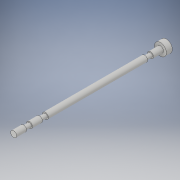
# Autodesk Inventor part: TornilloBasePixhawx
Saved by Autodesk Inventor 2019 (Build 230136000, 136)
## iProperties
Created: 2019-03-06
Part Number: TornilloBasePixhawx
Material: Generic
Document SubType Name: Modeling
Designer: Kenny
Density: 1 g/cm^3
Appearance: Default
Author: Kenny
Autodesk Inventor part; units mm, degrees
ref_plane "YZ Plane" through (0, 0, 0) normal (1, 0, 0) x (0, 1, 0)
ref_plane "XZ Plane" through (0, 0, 0) normal (0, 1, 0) x (-1, 0, 0)
ref_plane "XY Plane" through (0, 0, 0) normal (0, 0, 1) x (1, 0, 0)
sketch "Sketch1" plane through (0, 0, 0) normal (0, 0, 1) x (1, 0, 0)
  circle A0 centre (0, 0) radius 3
  dimension "d0" = 6
  constraints: 1 centre point, 1 coincident
  measures "d0" diameter of A0
extrude "Extrusion1" add sketch "Sketch1" along normal blind 3
sketch "Sketch5" plane through (0, 0, 3) normal (0, 0, 1) x (1, 0, 0)
  circle A0 centre (0, 0) radius 1.5
  dimension "d6" = 3
  constraints: 1 centre point, 1 coincident
  measures "d6" diameter of A0
extrude "Extrusion3" add sketch "Sketch5" along normal blind 5
sketch "Sketch6" plane through (0, 0, 8) normal (0, 0, 1) x (1, 0, 0)
  circle A0 centre (0, 0) radius 1
  dimension "d9" = 2
  constraints: 1 centre point, 1 coincident
  measures "d9" diameter of A0
extrude "Extrusion4" add sketch "Sketch6" along normal blind 3
sketch "Sketch7" plane through (0, 0, 11) normal (0, 0, 1) x (1, 0, 0)
  circle A0 centre (0, 0) radius 1 projected
  circle A1 centre (0, 0) radius 1.5
  dimension "d12" = 3
  constraints: 1 centre point, 1 coincident
  measures "d12" diameter of A1
extrude "Extrusion5" add sketch "Sketch7" along normal blind 50 contours A0 | A1
sketch "Sketch8" plane through (0, 0, 61) normal (0, 0, 1) x (1, 0, 0)
  circle A0 centre (0, 0) radius 1
  dimension "d15" = 2
  constraints: 1 centre point, 1 coincident
  measures "d15" diameter of A0
extrude "Extrusion6" add sketch "Sketch8" along normal blind 3
sketch "Sketch9" plane through (0, 0, 64) normal (0, 0, 1) x (1, 0, 0)
  circle A0 centre (0, 0) radius 1.5
  dimension "d18" = 3
  constraints: 1 centre point, 1 coincident
  measures "d18" diameter of A0
extrude "Extrusion7" add sketch "Sketch9" along normal blind 5
sketch "Sketch10" plane through (0, 0, 69) normal (0, 0, 1) x (1, 0, 0)
  circle A0 centre (0, 0) radius 1 projected
  circle A1 centre (0, 0) radius 1
  dimension "d21" = 2
  constraints: 1 centre point, 1 coincident
  measures "d21" diameter of A1
extrude "Extrusion8" add sketch "Sketch10" along normal blind 3
sketch "Sketch11" plane through (0, 0, 72) normal (0, 0, 1) x (1, 0, 0)
  circle A0 centre (0, 0) radius 1.5 projected
  circle A1 centre (0, 0) radius 1.5
  dimension "d24" = 3
  constraints: 1 centre point, 1 coincident
  measures "d24" diameter of A1
extrude "Extrusion9" add sketch "Sketch11" along normal blind 5
body "Solid1"
